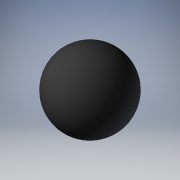
# Autodesk Inventor part: 60/28 Ball
Saved by Autodesk Inventor 2019 (Build 230136000, 136)
## iProperties
Created: 2024-02-20
Part Number: 60/28 Ball
Material: Generic
Catalog Web Link: www.cadenas.de
Description: Open type ball-Deep Groove Ball Bearings
Vendor: NTN
Document SubType Name: Modeling
Designer: psAdmin
Manufacturer: NTN
Mass: 0.185823 g
Surface Area: 1.57477 cm^2
Volume: 0.185823 cm^3
Density: 1 g/cm^3
Appearance: PSOLRGB-175-175-175
Category: PARTsolutions
Company: NTN
Title: 60/28 Ball
Author: Cadenas PARTsolutions
Comments: Deep Groove Ball Bearings
PSOL_IDENT_0: {$CADENAS_DATA/23d-libs/ntn/ball_roller_bearings/deep_groove_bb/deep_groove_bb/6_types/dgbb_ball.prj
PSOL_IDENT_1: },169 {VTYP=3D},{NB=60/28 Ball},{LINA=60/28 Ball},{NN=Open type ball},{DATE=17.10.2023 22:55:17},{GE
PSOL_IDENT_2: OMDATE=13.03.2020 06:49:14},{VERSION=},{LINEID=480},{WBVAR=},{WBNUMERIC=}  {NB=60/28 Ball},{LINA=60/
PSOL_IDENT_3: 28 Ball},{KT=DUMMY},{IDNR=},{SD=28},{D=52},{B=12},{R=0.6},{ORDER1=60/28},{ORDER=60/28},{CR=12.5},{CO
PSOL_IDENT_4: R=7.40},{CRF=1270},{CORF=755},{LSG=14000},{LSO=16000},{MASS=0.10},{RNS=0.5},{LLH=10000},{LLU=8400},{
PSOL_IDENT_5: ST=ZZ},{NCST=LLB},{LTST=LLH},{CST=LLU},{SRG=N},{SR=NR},{D1=49.73},{A=2.06},{BA=1.35},{R0=0.40},{D2=5
PSOL_IDENT_6: 7.9},{F=1.12},{DA1=32},{DA2=34},{DA=48},{DX=58.5},{CY=2.9},{CZ=1.2},{RAS=0.6},{RNAS=0.5},{VERS=1},{X=
PSOL_IDENT_7: 12}
NB: 60/28 Ball
NN: Open type ball
NT: Deep Groove Ball Bearings
NBSYN: $ORDER. Ball
LINA: 60/28 Ball
CATALOG: NTN Corporation
SD: 28
D: 52
B: 12
R: 0.6
ORDER1: 60/28
ORDER: 60/28
CR: 12.5
COR: 7.40
CRF: 1270
CORF: 755
LSG: 14000
LSO: 16000
MASS: 0.10
RNS: 0.5
LLH: 10000
LLU: 8400
ST: ZZ
NCST: LLB
LTST: LLH
CST: LLU
SRG: N
SR: NR
D1: 49.73
A: 2.06
BA: 1.35
R0: 0.4
D2: 57.9
F: 1.12
DA1: 32
DA2: 34
DA: 48
DX: 58.5
CY: 2.9
CZ: 1.2
RAS: 0.6
RNAS: 0.5
VERS: 1
SUPPLIER: NTN
ARTICLENO: 60/28 Ball
BOMINFO: 60/28 Ball
CREATOR: CADENAS GmbH
Autodesk Inventor part; units mm, degrees
sketch "Sketch_1" plane through (0, 0, 0) normal (0, 0, 1) x (1, 0, 0)
  line L0 (3.54, 0) -> (-3.54, 0)
  arc A0 (3.54, 0) -> (-3.54, 0) centre (0, 0) ccw
  line L1 (3.54, 0) -> (-3.54, 0)
  constraints: 4 end point, 2 point on circle, 1 centre point
revolve "Revolution1" add sketch "Sketch_1" angle 360 about axis through (3.54, 0, 0) along (1, 0, 0)
ref_plane "dgbb_ball_XY" through (0, 0, 0) normal (1, 0, 0) x (0, 0, -1)
ref_plane "dgbb_ball_YZ" through (0, 0, 0) normal (0, 0, -1) x (0, 1, 0)
ref_plane "dgbb_ball_ZX" through (0, 0, 0) normal (0, 1, 0) x (1, 0, 0)
body "Solid1"
